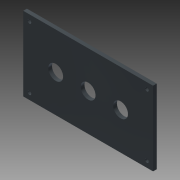
# Autodesk Inventor part: Front cover
Saved by Autodesk Inventor 2015 (Build 190159000, 159)
## iProperties
Created: 2015-09-07
Part Number: Front cover
Material: Iron, Gray
Document SubType Name: Modeling
Designer: Silas
Density: 7.15 g/cm^3
Appearance: Iron Gray
Mass: 127.251 g
Surface Area: 133.073 cm^2
Volume: 17.7973 cm^3
Author: Silas
Autodesk Inventor part; units mm, degrees
ref_plane "YZ Plane" through (0, 0, 0) normal (1, 0, 0) x (0, 1, 0)
ref_plane "XZ Plane" through (0, 0, 0) normal (0, 1, 0) x (-1, 0, 0)
ref_plane "XY Plane" through (0, 0, 0) normal (0, 0, 1) x (1, 0, 0)
sketch "Sketch1" plane through (0, 0, 0) normal (0, 1, 0) x (-1, 0, 0)
  line L0 (52.5, 30) -> (-52.5, 30)
  line L1 (-52.5, 30) -> (-52.5, -30)
  line L2 (-52.5, -30) -> (52.5, -30)
  line L3 (52.5, -30) -> (52.5, 30)
  line L4 (52.5, 0) -> (-52.5, 0) construction
  line L5 (0, 30) -> (0, -30) construction
  line L6 (0, 30) -> (52.5, 30) construction
  line L7 (26.25, 30) -> (26.25, -30) construction
  line L8 (0, 30) -> (-52.5, 30) construction
  line L9 (-26.25, 30) -> (-26.25, -30) construction
  circle A0 centre (26.25, 0) radius 6
  circle A1 centre (0, 0) radius 6
  circle A2 centre (-26.25, 0) radius 6
  line L10 (47.5, 25) -> (-47.5, 25) construction
  line L11 (-47.5, 25) -> (-47.5, -25) construction
  line L12 (-47.5, -25) -> (47.5, -25) construction
  line L13 (47.5, -25) -> (47.5, 25) construction
  circle A3 centre (47.5, 25) radius 1.5
  circle A4 centre (47.5, -25) radius 1.5
  circle A5 centre (-47.5, -25) radius 1.5
  circle A6 centre (-47.5, 25) radius 1.5
  dimension "d0" = 105
  dimension "d1" = 60
  dimension "d2" = 12
  dimension "d3" = 12
  dimension "d4" = 12
  dimension "d5" = 5
  dimension "d6" = 3
  dimension "d7" = 3
  dimension "d8" = 3
  dimension "d9" = 3
  constraints: 28 end point, 9 midpoint, 7 centre point, 6 coincident, 5 perpendicular, 4 parallel, 2 point on line, 1 collinear, 1 horizontal, 3 other
  measures "d0" distance of L0.start L0.end
  measures "d1" distance of L2.end L0.start
  measures "d2" diameter of A0
  measures "d3" diameter of A1
  measures "d4" diameter of A2
  measures "d5" distance between parallel lines of L3 L13
  measures "d6" diameter of A3
  measures "d7" diameter of A4
  measures "d8" diameter of A5
  measures "d9" diameter of A6
extrude "Extrusion1" add sketch "Sketch1" along normal blind 3
body "Solid1"
